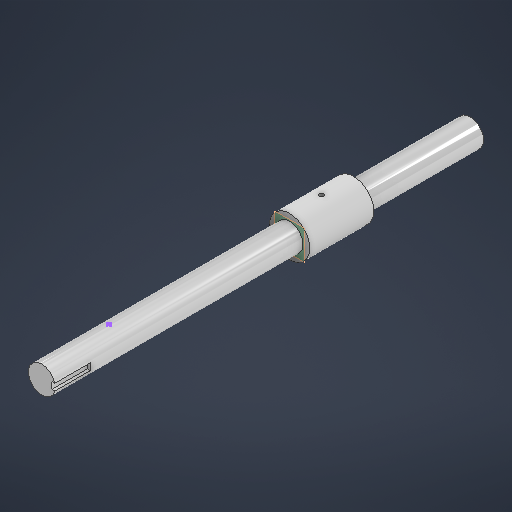
# Autodesk Inventor part: Rough draft shaft
Saved by Autodesk Inventor 2026.3 (Build 303398000, 398)
## iProperties
Created: 2026-07-22
Part Number: Rough draft shaft
Material: Generic
Document SubType Name: Sheet Metal
Designer: matot
Density: 1 g/cm^3
Sheet Metal Rule: Default_mm
Appearance: Default
Author: matot
Autodesk Inventor part; units mm, degrees
ref_plane "YZ Plane" through (0, 0, 0) normal (1, 0, 0) x (0, 1, 0)
ref_plane "XZ Plane" through (0, 0, 0) normal (0, 1, 0) x (-1, 0, 0)
ref_plane "XY Plane" through (0, 0, 0) normal (0, 0, 1) x (1, 0, 0)
sketch "Sketch1" plane through (0, 0, 0) normal (0, 0, 1) x (1, 0, 0)
  circle A0 centre (0, 0) radius 10
  dimension "d0" = 20
  constraints: 1 centre point, 1 coincident
  measures "d0" diameter of A0
extrude "Extrusion1" add sketch "Sketch1" along normal blind 65
sketch "Sketch2" plane through (0, 0, 65) normal (0, 0, 1) x (1, 0, 0)
  circle A0 centre (0, 0) radius 10
  dimension "d3" = 20
  constraints: 1 centre point, 1 coincident
  measures "d3" diameter of A0
extrude "Extrusion2" add sketch "Sketch2" along normal blind 150
sketch "Sketch3" plane through (0, 0, 0) normal (0, 0, -1) x (-1, 0, 0)
  circle A0 centre (0, 0) radius 10
  constraints: 1 centre point, 1 coincident
extrude "Extrusion3" add sketch "Sketch3" along normal blind 100
sketch "Sketch4" plane through (0, 0, 215) normal (0, 0, 1) x (1, 0, 0)
  point P0 (0, 0)
  point P1 (0, 10)
ref_plane "Work Plane1" through (0, 10, 215) normal (0, 1, 0) x (-1, 0, 0)
sketch "Sketch5" plane through (0, 10, 215) normal (0, 1, 0) x (-1, 0, 0)
  line L0 (10, 0) -> (-10, 0) projected
  circle A0 centre (0, -157.5) radius 2
  point P0 (0, -215)
  dimension "d8" = 157.5
  dimension "d9" = 4
  constraints: 1 centre point, 1 coincident
  measures "d8" distance from line of point (0, -157.5) L0
  measures "d9" diameter of A0
hole "Hole1" at (0, 10, 57.5) direction (0, -1, 0) diameter 3.242 end through all thread size "M4x0.7" class "6H" standard "ISO Metric profile"
sketch "Sketch6" plane through (0, 0, -100) normal (0, 0, -1) x (-1, 0, 0)
  circle A0 centre (0, 0) radius 10
  constraints: 1 centre point, 1 coincident
extrude "Extrusion4" cut sketch "Sketch6" against normal blind 54
sketch "Sketch7" plane through (0, 0, 215) normal (0, 0, 1) x (1, 0, 0)
  circle A0 centre (0, 0) radius 10
  constraints: 1 centre point, 1 coincident
extrude "Extrusion5" add sketch "Sketch7" along normal blind 50
ref_plane "Work Plane3" through (0, 0, 81) normal (0, 0, -1) x (-1, 0, 0)
sketch "Sketch9" plane through (0, 0, 81) normal (0, 0, -1) x (-1, 0, 0)
  circle A0 centre (0, 0) radius 15
  dimension "d29" = 30
  constraints: 1 centre point, 1 coincident
  measures "d29" diameter of A0
extrude "Extrusion7" add sketch "Sketch9" along normal blind 47.6
sketch "Sketch10" plane through (0, 10, 215) normal (0, 1, 0) x (-1, 0, 0)
  line L0 (-15, -134) -> (15, -134) projected
  point P0 (0, -215)
  point P1 (0, -157.8)
  dimension "d32" = 23.8
  measures "d32" distance from line of point (0, -157.8) L0
hole "Hole2" at (0, 10, 57.2) direction (0, -1, 0) diameter 3.4587 end through all thread size "M4x0.5" class "6H" standard "ISO Metric profile"
sketch "Sketch11" plane through (0, 10, 57.2) normal (0, -1, 0) x (1, 0, 0)
  point P0 (0, -57.2)
  point P1 (0, 0)
hole "Hole3" at (0, 10, 57.2) direction (0, 1, 0) diameter 3.4587 end through all thread size "M4x0.5" class "6H" standard "ISO Metric profile"
sketch "Sketch12" plane through (0, 0, -46) normal (0, 0, -1) x (-1, 0, 0)
  circle A0 centre (0, 0) radius 10
  constraints: 1 centre point, 1 coincident
extrude "Extrusion8" add sketch "Sketch12" along normal blind 7.2
sketch "Sketch15" plane through (0, 0, 265) normal (0, 0, 1) x (1, 0, 0)
  line L0 (10, 2.5) -> (7.5, 2.5)
  line L1 (7.5, 2.5) -> (7.5, -2.5)
  line L2 (7.5, -2.5) -> (10, -2.5)
  line L3 (10, -2.5) -> (10, 2.5)
  point P0 (0, 0)
  point P1 (8.75, -2.5)
  dimension "d62" = 5
  dimension "d63" = 10
  dimension "d64" = 2.5
  constraints: 8 end point, 2 parallel, 1 horizontal, 1 midpoint, 1 perpendicular
  measures "d62" distance of L0.end L1.end
  measures "d63" distance from line of point (0, 0) L3
  measures "d64" vertical distance of point (0, 0) point (8.75, -2.5)
extrude "Extrusion11" cut sketch "Sketch15" against normal blind 26.4
equation "\"d15\" = Thickness"
equation "\"d38\" = Thickness"
equation "\"BendRadius\" = Thickness"
equation "\"BendReliefWidth\" = Thickness"
equation "\"BendReliefDepth\" = 0.5 * Thickness"
equation "\"CornerReliefSize\" = 4 * Thickness"
equation "\"MinimumRemnant\" = 2 * Thickness"
equation "\"TransitionRadius\" = BendRadius"
equation "\"JacobiRadiusSize\" = BendRadius"
equation "\"GapSize\" = Thickness"
equation "\"Thickness\" = 0.5"
body "Solid1"
